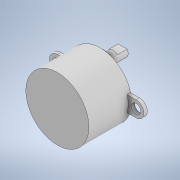
# Autodesk Inventor part: motooor
Saved by Autodesk Inventor 2022 (Build 260153000, 153)
## iProperties
Created: 2022-08-28
Part Number: motooor
Material: Generic
Document SubType Name: Modeling
Designer: Ruslana Zubareva
Density: 1 g/cm^3
Appearance: Default
Author: Ruslana Zubareva
Autodesk Inventor part; units mm, degrees
ref_plane "YZ Plane" through (0, 0, 0) normal (1, 0, 0) x (0, 1, 0)
ref_plane "XZ Plane" through (0, 0, 0) normal (0, 1, 0) x (-1, 0, 0)
ref_plane "XY Plane" through (0, 0, 0) normal (0, 0, 1) x (1, 0, 0)
sketch "Sketch1" plane through (0, 0, 0) normal (0, 0, 1) x (1, 0, 0)
  circle A0 centre (0, 0) radius 14
  line L0 (0, 14) -> (0, -14)
  line L1 (-17.5, 9.3538) -> (-17.5, -9.6398)
  circle A1 centre (-17.5, 0) radius 2.1
  arc A2 (-17.5, 3.5) -> (-17.5, -3.5) centre (-17.5, 0) ccw
  line L2 (-17.5, 3.5) -> (-13.5554, 3.5)
  line L3 (-17.5, -3.5) -> (-13.5554, -3.5)
  dimension "d0" = 28
  dimension "d1" = 17.5
  dimension "d2" = 4.2
  dimension "d5" = 7
  constraints: 8 end point, 6 point on circle, 3 centre point, 3 coincident, 3 point on line, 2 perpendicular, 2 tangent, 2 vertical, 1 horizontal alignment, 1 midpoint
  measures "d0" diameter of A0
  measures "d1" distance between parallel lines of L0 L1
  measures "d2" diameter of A1
  measures "d5" diameter of A2
extrude "Extrusion1" add sketch "Sketch1" along normal blind 19 contours A0 L0 | L0 A0
extrude "Extrusion2" add sketch "Sketch1" along normal blind 1.5 contours A0 L3 L1 A1 L2 | L1 A1 A2
mirror "Mirror1" about plane through (0, 0, 0) normal (1, 0, 0) of "Extrusion2"
sketch "Sketch3" plane through (0, 0, 0) normal (0, 0, -1) x (-1, 0, 0)
  circle A0 centre (0, 8) radius 4.5
  circle A1 centre (0, 8) radius 2.5
  line L0 (-2, 9.5) -> (2, 9.5)
  line L1 (-2, 6.5) -> (2, 6.5)
  point P0 (0, 0)
  point P1 (0, 10.5)
  point P2 (0, 5.5)
  dimension "d8" = 9
  dimension "d9" = 8
  dimension "d10" = 5
  dimension "d12" = 1
  dimension "d13" = 1
  constraints: 6 point on circle, 4 end point, 3 vertical alignment, 2 centre point, 2 horizontal, 1 coincident
  measures "d8" diameter of A0
  measures "d9" distance of point (0, 0) A0.centre
  measures "d10" diameter of A1
  measures "d12" distance from line of point (0, 10.5) L0
  measures "d13" distance from line of L1 point (0, 5.5)
extrude "Extrusion3" add sketch "Sketch3" along normal blind 1.5 contours A0 | A1 L1 L0 | L0 A1 | A1 L1
extrude "Extrusion4" add sketch "Sketch3" along normal blind 5.5 contours A1 L1 L0 | L0 A1 | A1 L1
extrude "Extrusion5" add sketch "Sketch3" along normal blind 10 contours A1 L1 L0
body "Solid1"
